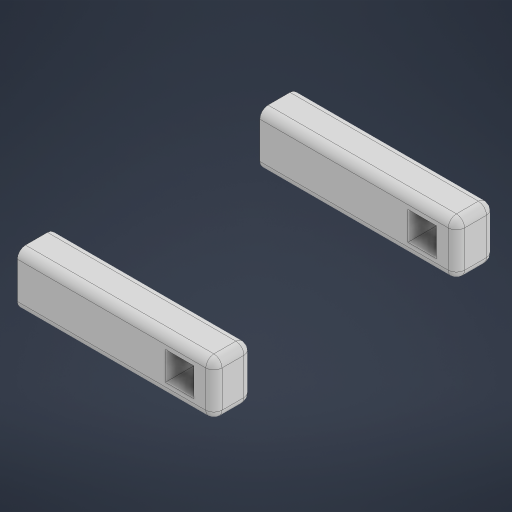
# Autodesk Inventor part: clamp
Saved by Autodesk Inventor 2024.4 (Build 284460000, 460)
## iProperties
Created: 2026-02-18
Part Number: clamp
Material: Ogólny
Document SubType Name: Modeling
Designer: User
Density: 1 g/cm^3
Appearance: Domyślna
Author: User
Autodesk Inventor part; units mm, degrees
ref_plane "YZ Plane" through (0, 0, 0) normal (1, 0, 0) x (0, 1, 0)
ref_plane "XZ Plane" through (0, 0, 0) normal (0, 1, 0) x (-1, 0, 0)
ref_plane "XY Plane" through (0, 0, 0) normal (0, 0, 1) x (1, 0, 0)
sketch "Szkic1" plane through (0, 0, 0) normal (0, 1, 0) x (-1, 0, 0)
  line L0 (-19.3, 25.1) -> (19.3, 25.1)
  line L1 (19.3, 25.1) -> (19.3, -25.1)
  line L2 (19.3, -25.1) -> (-19.3, -25.1)
  line L3 (-19.3, -25.1) -> (-19.3, 25.1)
  line L4 (-19.3, 25.1) -> (19.3, -25.1) construction
  line L5 (19.3, 25.1) -> (-19.3, -25.1) construction
  line L6 (-29, 34.5) -> (29, 34.5)
  line L7 (29, 34.5) -> (29, -34.5)
  line L8 (29, -34.5) -> (-29, -34.5)
  line L9 (-29, -34.5) -> (-29, 34.5)
  line L10 (-29, 34.5) -> (29, -34.5) construction
  line L11 (29, 34.5) -> (-29, -34.5) construction
  line L12 (19.3, 25.1) -> (19.3, 34.5)
  line L13 (19.3, -25.1) -> (19.3, -34.5)
  line L14 (-19.3, 25.1) -> (-29, 25.1)
  line L15 (-19.3, -25.1) -> (-29, -25.1)
  point P0 (0, 0)
  dimension "d0" = 38.6
  dimension "d1" = 50.2
  dimension "d2" = 58
  dimension "d3" = 69
  constraints: 32 end point, 5 perpendicular, 4 midpoint, 4 parallel, 4 point on line, 2 horizontal, 1 vertical
  measures "d0" distance of L1.end L2.end
  measures "d1" distance of L0.end L1.end
  measures "d2" distance of L7.end L8.end
  measures "d3" distance of L6.end L7.end
extrude "Wyciągnięcie proste1" add sketch "Szkic1" along normal blind 13 contours L14 L9 L6 L12 L0 | L2 L13 L8 L9 L15
sketch "Szkic2" plane through (-19.3, 0, 25.1) normal (-1, 0, 0) x (0, 0, 1)
  line L0 (9.4, 0) -> (-59.6, 0) projected
  line L1 (9.4, 0) -> (-59.6, 0)
  line L2 (-25.1, 0) -> (-25.1, 13)
  line L3 (-50.2, 13) -> (0, 13) projected
  line L4 (0, 0) -> (0, 13) projected
  line L5 (9.4, 0) -> (0, 0)
  line L6 (4.7, 0) -> (4.7, 13)
  line L7 (9.4, 13) -> (-59.6, 13) projected
  circle A0 centre (4.7, 6.5) radius 2.6
  circle A1 centre (-54.9, 6.5) radius 2.6
  dimension "d6" = 5.2
  constraints: 8 end point, 3 midpoint, 2 centre point, 1 horizontal, 1 perpendicular, 1 point on line, 1 symmetric about line, 1 vertical, 1 other
  measures "d6" diameter of A0
extrude "Wyciągnięcie proste2" cut sketch "Szkic2" against normal blind 10 contours A0 L6 | L6 A0 | A1
sketch "Szkic3" plane through (-19.3, 0, 34.5) normal (0, 0, 1) x (1, 0, 0)
  line L0 (48.3, 0) -> (48.3, 13) projected
  line L1 (48.3, 0) -> (48.3, 13)
  line L2 (48.3, 13) -> (48.3, 6.5)
  line L3 (48.3, 6.5) -> (39.9, 6.5)
  line L4 (48.3, 6.5) -> (56.7, 6.5) construction
  line L5 (43.4, 3) -> (36.4, 3)
  line L6 (36.4, 3) -> (36.4, 10)
  line L7 (36.4, 10) -> (43.4, 10)
  line L8 (43.4, 10) -> (43.4, 3)
  line L9 (43.4, 3) -> (36.4, 10) construction
  line L10 (36.4, 3) -> (43.4, 10) construction
  point P0 (19.3, 0)
  dimension "d10" = 8.4
  dimension "d11" = 180
  dimension "d12" = 7
  dimension "d13" = 7
  constraints: 20 end point, 3 equal length, 3 horizontal, 3 midpoint, 1 collinear, 1 perpendicular
  measures "d10" distance of L2.end L3.end
  measures "d11" angle of L3 L4
  measures "d12" distance of L6.end L7.end
  measures "d13" distance of L5.end L6.end
extrude "Wyciągnięcie proste3" cut sketch "Szkic3" against normal blind 98.25
fillet "Zaokrąglenie2" radius 2 16 edges at (29, 13, 29.8) (29, 0, 29.8) (29, 0, -29.8) (29, 13, -29.8) (4.85, 13, -34.5) (4.85, 13, 34.5) (4.85, 0, 34.5) (4.85, 0, -34.5) (4.85, 13, 25.1) (4.85, 0, 25.1) (4.85, 0, -25.1) (4.85, 13, -25.1) (29, 6.5, 34.5) (29, 6.5, 25.1) (29, 6.5, -25.1) (29, 6.5, -34.5)
